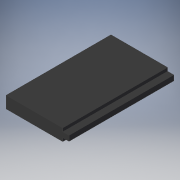
# Autodesk Inventor part: Maze Wall Middle
Saved by Autodesk Inventor 2019 (Build 230136000, 136)
## iProperties
Created: 2019-01-23
Part Number: Maze Wall Middle
Material: Generic
Document SubType Name: Modeling
Designer: Billy
Density: 1 g/cm^3
Appearance: Default
Author: Billy
Autodesk Inventor part; units mm, degrees
ref_plane "YZ Plane" through (0, 0, 0) normal (1, 0, 0) x (0, 1, 0)
ref_plane "XZ Plane" through (0, 0, 0) normal (0, 1, 0) x (-1, 0, 0)
ref_plane "XY Plane" through (0, 0, 0) normal (0, 0, 1) x (1, 0, 0)
sketch "Sketch1" plane through (0, 0, 0) normal (0, 1, 0) x (-1, 0, 0)
  line L0 (0, 0) -> (30, 0)
  line L1 (30, 0) -> (30, -50)
  line L2 (30, -50) -> (0, -50)
  line L3 (0, -50) -> (0, 0)
  dimension "d0" = 30
  dimension "d1" = 50
  constraints: 8 end point, 2 parallel, 1 horizontal, 1 perpendicular
  measures "d0" distance of L1.end L2.end
  measures "d1" distance of L0.end L1.end
extrude "Extrusion1" add sketch "Sketch1" along normal blind 5.65
sketch "Sketch2" plane through (-30, 0, 0) normal (0, 0, 1) x (1, 0, 0)
  line L0 (30, 0) -> (0, 0) projected
  line L1 (30, 0) -> (30, 5.65) projected
  line L2 (0, 5.65) -> (30, 5.65) projected
  line L3 (0, 0) -> (0, 5.65) projected
  line L4 (30, 0) -> (0, 0) projected
  line L5 (30, 0) -> (27, 0)
  line L6 (27, 0) -> (27, 1.5)
  line L7 (27, 1.5) -> (30, 1.5)
  line L8 (30, 1.5) -> (30, 0)
  line L9 (30, 5.65) -> (27, 5.65)
  line L10 (27, 5.65) -> (27, 4.15)
  line L11 (27, 4.15) -> (30, 4.15)
  line L12 (30, 4.15) -> (30, 5.65)
  dimension "d4" = 3
  dimension "d5" = 1.5
  dimension "d6" = 3
  dimension "d7" = 1.5
  constraints: 16 end point, 4 parallel, 2 horizontal, 2 perpendicular
  measures "d4" distance of L6.end L7.end
  measures "d5" distance of L5.end L6.end
  measures "d6" distance of L11.end L10.end
  measures "d7" distance of L10.end L9.end
extrude "Extrusion2" cut sketch "Sketch2" against normal up to surface (50 mm away) contours L0 L6 L7 L1 | L11 L10 L2 L1
move faces "Move1" translate (0, -0.1, 0) faces at (-2, 4.15, -16.6667)
move faces "Move2" translate (0, 0.1, 0) faces at (-1, 1.5, -16.6667)
body "Solid1"
